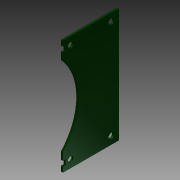
# Autodesk Inventor part: PCBModuleRight01
Saved by Autodesk Inventor 2013 (Build 170138000, 138)
## iProperties
Created: 2014-07-14
Part Number: PCBModuleRight01
Material: PCB(1)
Document SubType Name: Modeling
Designer: spichelh
Density: 1 g/cm^3
Author: spichelh
Autodesk Inventor part; units mm, degrees
ref_plane "YZ Plane" through (0, 0, 0) normal (1, 0, 0) x (0, 1, 0)
ref_plane "XZ Plane" through (0, 0, 0) normal (0, 1, 0) x (-1, 0, 0)
ref_plane "XY Plane" through (0, 0, 0) normal (0, 0, 1) x (1, 0, 0)
sketch "Sketch1" plane through (0, 0, 0) normal (1, 0, 0) x (0, 1, 0)
  line L0 (0, 0) -> (57.15, 0)
  line L1 (57.15, 0) -> (57.15, 27.94)
  line L2 (0, 0) -> (0, 27.94)
  arc A0 (8.89, 27.94) -> (48.26, 27.94) centre (28.575, 49.4224) ccw
  line L3 (28.575, 0) -> (28.575, 8.5438) construction
  circle A1 centre (3.81, 3.81) radius 1.4
  circle A2 centre (53.34, 3.81) radius 1.4
  line L4 (0, 27.94) -> (2.54, 27.94)
  line L5 (2.54, 27.94) -> (2.54, 26.67)
  line L6 (2.54, 26.67) -> (5.08, 26.67)
  line L7 (5.08, 26.67) -> (5.08, 27.94)
  line L8 (5.08, 27.94) -> (8.89, 27.94)
  line L9 (57.15, 27.94) -> (54.61, 27.94)
  line L10 (54.61, 27.94) -> (54.61, 26.67)
  line L11 (54.61, 26.67) -> (52.07, 26.67)
  line L12 (52.07, 26.67) -> (52.07, 27.94)
  line L13 (52.07, 27.94) -> (48.26, 27.94)
  circle A3 centre (53.34, 24.13) radius 1.4
  circle A4 centre (3.81, 24.13) radius 1.4
  dimension "d0" = 57.15
  dimension "d1" = 27.94
  dimension "d2" = 27.94
  dimension "d3" = 85
  dimension "d4" = 29.1375
  dimension "d5" = 2.8
  dimension "d6" = 3.81
  dimension "d7" = 3.81
  dimension "d8" = 2.54
  dimension "d9" = 1.27
  dimension "d10" = 2.54
  dimension "d11" = 1.27
  dimension "d14" = 2.8
  dimension "d15" = 20.32
  constraints: 28 end point, 6 symmetric about line, 5 centre point, 4 perpendicular, 3 parallel, 2 horizontal alignment, 2 point on circle, 1 horizontal, 1 midpoint, 1 point on line, 1 vertical alignment, 2 other
  measures "d0" distance of L0.start L0.end
  measures "d1" distance of L0.end L1.end
  measures "d2" distance of L0.start L2.end
  measures "d4" radius of A0
  measures "d5" diameter of A1
  measures "d6" distance from line of L0 A1.centre
  measures "d7" distance from line of L2 A1.centre
  measures "d8" distance of L2.end L4.end
  measures "d9" distance of L4.end L5.end
  measures "d10" distance of L5.end L6.end
  measures "d11" distance of L6.end L7.end
  measures "d14" diameter of A3
  measures "d15" distance of A2.centre A3.centre
extrude "Extrusion1" add sketch "Sketch1" along normal blind 1
body "Solid1"
